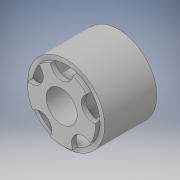
# Autodesk Inventor part: wheel
Saved by Autodesk Inventor 2016 (Build 200138000, 138)
## iProperties
Created: 2016-01-14
Part Number: wheel
Material: Generic
Document SubType Name: Modeling
Designer: 126612
Density: 1 g/cm^3
Appearance: Default
Author: 126612
Autodesk Inventor part; units mm, degrees
ref_plane "YZ Plane" through (0, 0, 0) normal (1, 0, 0) x (0, 1, 0)
ref_plane "XZ Plane" through (0, 0, 0) normal (0, 1, 0) x (-1, 0, 0)
sketch "Sketch1" plane through (0, 0, 0) normal (0, 0, 1) x (1, 0, 0)
  circle A0 centre (0, 0) radius 10.668
  circle A1 centre (0, 0) radius 9.398
  circle A2 centre (0, 0) radius 5.588
  circle A3 centre (0, 0) radius 4.318
  dimension "d0" = 21.336
  dimension "d1" = 1.27
  dimension "d2" = 11.176
  dimension "d3" = 1.27
  constraints: 4 centre point, 4 coincident
  measures "d0" diameter of A0
  measures "d1" radial gap between concentric circles of A0 A1
  measures "d2" diameter of A2
  measures "d3" radial gap between concentric circles of A2 A3
extrude "Extrusion1" add sketch "Sketch1" along normal blind 14.478
ref_plane "Work Plane1" through (0, 0, 7.239) normal (0, 0, 1) x (1, 0, 0)
sketch "Sketch2" plane through (0, 0, 14.478) normal (0, 0, 1) x (1, 0, 0)
  circle A0 centre (0, 0) radius 9.398
  circle A1 centre (0, 0) radius 10.668 projected
  dimension "d6" = 1.27
  constraints: 1 centre point, 1 coincident
  measures "d6" radial gap between concentric circles of A1 A0
extrude "Extrusion2" add sketch "Sketch2" along normal blind 1.27 contours A0
sketch "Sketch3" plane through (0, 0, 15.748) normal (0, 0, 1) x (1, 0, 0)
  circle A0 centre (0, 0) radius 4.318
  constraints: 1 centre point, 1 coincident
extrude "Extrusion3" cut sketch "Sketch3" against normal blind 1.27
sketch "Sketch4" plane through (0, 0, 15.748) normal (0, 0, 1) x (1, 0, 0)
  circle A0 centre (0, 0) radius 9.398 projected
  circle A1 centre (0, 9.398) radius 3.175
  dimension "d11" = 6.35
  constraints: 1 centre point, 1 vertical alignment, 1 other
  measures "d11" diameter of A1
extrude "Extrusion4" cut sketch "Sketch4" against normal blind 1.27 contours A1 A0 | A0 A1 picked at (0, 8.2996) picked at (-0.0897, 10.4125)
sketch "Sketch5" plane through (0, 0, 15.748) normal (0, 0, 1) x (1, 0, 0)
  circle A0 centre (0, 0) radius 9.398 projected
  circle A1 centre (5.9392, -7.2834) radius 3.175
  dimension "d14" = 6.35
  constraints: 1 centre point, 2 other
  measures "d14" diameter of A1
extrude "Extrusion5" cut sketch "Sketch5" against normal blind 1.27 contours A1 A0 | A0 A1 picked at (5.2451, -6.4322) picked at (6.5249, -8.1165)
sketch "Sketch6" plane through (0, 0, 15.748) normal (0, 0, 1) x (1, 0, 0)
  arc A0 (-3.1294, 8.8617) -> (3.1751, -8.8454) centre (0, 0) ccw projected
  circle A1 centre (-5.9223, -7.2972) radius 3.175
  dimension "d17" = 6.35
  constraints: 1 centre point, 1 point on circle
  measures "d17" diameter of A1
extrude "Extrusion6" cut sketch "Sketch6" against normal blind 1.27
sketch "Sketch7" plane through (0, 0, 15.748) normal (0, 0, 1) x (1, 0, 0)
  circle A0 centre (0, 0) radius 9.398 projected
  circle A1 centre (-8.278, 4.4494) radius 3.175
  dimension "d20" = 6.35
  constraints: 1 centre point, 2 other
  measures "d20" diameter of A1
extrude "Extrusion7" cut sketch "Sketch7" against normal blind 1.27 contours A1 A0 | A0 A1 picked at (-7.3008, 3.9478) picked at (-9.1749, 4.9315)
sketch "Sketch8" plane through (0, 0, 15.748) normal (0, 0, 1) x (1, 0, 0)
  arc A0 (8.0256, -4.8901) -> (3.1294, 8.8617) centre (0, 0) ccw projected
  circle A1 centre (8.6453, 3.6853) radius 3.175
  dimension "d23" = 6.35
  constraints: 1 centre point, 1 point on circle
  measures "d23" diameter of A1
extrude "Extrusion8" cut sketch "Sketch8" against normal blind 1.27
body "Solid1"
